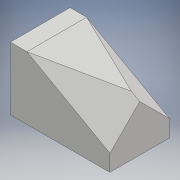
# Autodesk Inventor part: 8
Saved by Autodesk Inventor 2017 (Build 210142000, 142)
## iProperties
Part Number: 8
Material: 一般
Document SubType Name: Modeling
Designer: Brian
Density: 1 g/cm^3
Appearance: 預設
Mass: 68.22 g
Surface Area: 100.581 cm^2
Volume: 68.22 cm^3
Author: Brian
Autodesk Inventor part; units mm, degrees
ref_plane "YZ Plane" through (0, 0, 0) normal (1, 0, 0) x (0, 1, 0)
ref_plane "XZ Plane" through (0, 0, 0) normal (0, 1, 0) x (-1, 0, 0)
sketch "草圖1" plane through (0, 0, 0) normal (0, 1, 0) x (-1, 0, 0)
  line L0 (0, 0) -> (-60, 0)
  line L1 (-60, 0) -> (-60, -38)
  line L2 (-60, -38) -> (0, -38)
  line L3 (0, -38) -> (0, 0)
  dimension "d0" = 60
  dimension "d1" = 38
  constraints: 8 end point, 2 parallel, 1 horizontal, 1 perpendicular
  measures "d0" distance of L1.end L2.end
  measures "d1" distance of L2.end L0.start
extrude "擠出1" add sketch "草圖1" along normal mid plane 36
sketch "草圖2" plane through (0, 18, 0) normal (0, 1, 0) x (1, 0, 0)
  line L0 (0, 0) -> (60, 0) projected
  line L1 (10, 0) -> (60, 8)
  line L2 (60, 0) -> (60, 38) projected
  dimension "d4" = 10
  dimension "d5" = 30
  constraints: 2 end point, 2 point on line
  measures "d4" distance of L0.start L1.start
  measures "d5" distance of L2.end L1.end
extrude "擠出2" cut sketch "草圖2" against normal blind 40
sketch "草圖3" plane through (60, -18, -38) normal (1, 0, 0) x (0, 0, -1)
  line L0 (-30, 16) -> (-10, 36)
  line L1 (0, 36) -> (-38, 36) projected
  line L2 (-30, 36) -> (-30, 0) projected
  point P0 (-38, 18)
  dimension "d8" = 20
  dimension "d9" = 20
  constraints: 2 end point, 2 point on line
  measures "d8" horizontal distance of L0.start L0.end
  measures "d9" horizontal distance of L0.start L0.end
ref_plane "工作平面1" through (10, 18, 0) normal (-0.3682, -0.6574, -0.6574) x (0.8725, 0, -0.4886)
sketch "草圖4" plane through (10, 18, 0) normal (-0.3682, -0.6574, -0.6574) x (0.8725, 0, -0.4886)
  line L0 (-15.1543, -12.3218) -> (93.717, -12.3218)
  line L1 (93.717, -12.3218) -> (93.717, 28.8166)
  line L2 (93.717, 28.8166) -> (-15.1543, 28.8166)
  line L3 (-15.1543, 28.8166) -> (-15.1543, -12.3218)
  point P0 (-8.7251, 10.3509)
  constraints: 8 end point, 2 parallel, 1 horizontal, 1 perpendicular
extrude "擠出3" cut sketch "草圖4" against normal blind 40
mirror "鏡射1" about plane through (0, 0, 0) normal (0, 1, 0) of "擠出3"
